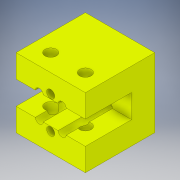
# Autodesk Inventor part: sevo_piece
Saved by Autodesk Inventor 2019 (Build 230136000, 136)
## iProperties
Created: 2019-02-02
Part Number: sevo_piece
Material: Generic
Document SubType Name: Modeling
Designer: suchanek
Density: 1 g/cm^3
Appearance: Default
Author: suchanek
Autodesk Inventor part; units mm, degrees
ref_plane "YZ Plane" through (0, 0, 0) normal (1, 0, 0) x (0, 1, 0)
ref_plane "XZ Plane" through (0, 0, 0) normal (0, 1, 0) x (-1, 0, 0)
ref_plane "XY Plane" through (0, 0, 0) normal (0, 0, 1) x (1, 0, 0)
sketch "Sketch1" plane through (0, 0, 0) normal (0, 0, 1) x (1, 0, 0)
  circle A0 centre (0, 0) radius 10
  circle A1 centre (0, 7) radius 0.85
  circle A2 centre (-4.9497, 4.9497) radius 0.85
  circle A3 centre (-7, 0) radius 0.85
  circle A4 centre (-4.9497, -4.9497) radius 0.85
  circle A5 centre (0, -7) radius 0.85
  circle A6 centre (4.9497, -4.9497) radius 0.85
  circle A7 centre (7, 0) radius 0.85
  circle A8 centre (4.9497, 4.9497) radius 0.85
  dimension "d0" = 20
  dimension "d1" = 7
  dimension "d2" = 1.7
  dimension "d5" = 360
  constraints: 9 centre point, 2 coincident, 1 vertical alignment, 17 other
  measures "d0" diameter of A0
  measures "d1" distance of A1.centre point (0, 0)
  measures "d2" diameter of A1
extrude "Extrusion1" add sketch "Sketch1" along normal blind 14
sketch "Sketch2" plane through (0, 0, 14) normal (0, 0, 1) x (1, 0, 0)
  line L0 (15, -15) -> (-15, -15)
  line L1 (-15, -15) -> (-15, 15)
  line L2 (-15, 15) -> (15, 15)
  line L3 (15, 15) -> (15, -15)
  line L4 (15, -15) -> (-15, 15) construction
  line L5 (-15, -15) -> (15, 15) construction
  point P0 (0, 0)
  dimension "d9" = 30
  dimension "d10" = 30
  constraints: 12 end point, 2 midpoint, 2 parallel, 1 horizontal, 1 perpendicular
  measures "d9" distance of L1.end L2.end
  measures "d10" distance of L0.end L1.end
extrude "Extrusion2" add sketch "Sketch2" against normal blind 10
sketch "Sketch3" plane through (0, 0, 14) normal (0, 0, 1) x (1, 0, 0)
  line L0 (15, 15) -> (15, -15) projected
  line L1 (-15, -15) -> (15, -15)
  line L2 (15, -15) -> (15, -5.1)
  line L3 (15, -5.1) -> (-15, -5.1)
  line L4 (-15, -5.1) -> (-15, -15)
  line L5 (-15, -15) -> (-15, 15) projected
  line L6 (15, 15) -> (-15, 15)
  line L7 (-15, 15) -> (-15, 5.1)
  line L8 (-15, 5.1) -> (15, 5.1)
  line L9 (15, 5.1) -> (15, 15)
  point P0 (0, 0)
  dimension "d13" = 9.9
  dimension "d14" = 9.9
  constraints: 16 end point, 4 parallel, 2 horizontal, 2 perpendicular, 2 point on line
  measures "d13" distance between parallel lines of L1 L3
  measures "d14" distance between parallel lines of L6 L8
extrude "Extrusion3" add sketch "Sketch3" along normal blind 20 contours L0 L8 L5 L6 | L0 L1 L4 L3
sketch "Sketch4" plane through (0, 0, 14) normal (0, 0, 1) x (1, 0, 0)
  point P0 (0, 0)
  point P1 (7, 0)
  point P2 (4.9497, 4.9497)
  point P3 (0, 7)
  point P4 (-4.9497, 4.9497)
  point P5 (-7, 0)
  point P6 (-4.9497, -4.9497)
  point P7 (0, -7)
  point P8 (4.9497, -4.9497)
  dimension "d17" = 7
  dimension "d20" = 360
  constraints: 1 horizontal alignment, 9 other
  measures "d17" distance of point (0, 0) point (7, 0)
hole "Hole1" at (0, -7, 14) at (-4.9497, -4.9497, 14) at (-7, 0, 14) at (4.9497, -4.9497, 14) at (4.9497, 4.9497, 14) at (7, 0, 14) at (-4.9497, 4.9497, 14) at (0, 7, 14) direction (0, 0, -1) diameter 1.8 depth 10 start extended yes counterbore diameter 3.5 counterbore depth 2
sketch "Sketch5" plane through (-15, 15, 4) normal (0, 1, 0) x (1, 0, 0)
  circle A0 centre (7.5, -22.5) radius 2.5
  circle A1 centre (22.5, -22.5) radius 2.5
  line L0 (15, 4) -> (15, -14.6414)
  line L1 (0, -30) -> (0, 0) projected
  line L2 (0, 0) -> (30, 0) projected
  dimension "d29" = 5
  dimension "d30" = 5
  dimension "d32" = 15
  dimension "d33" = 22.5
  constraints: 2 centre point, 2 end point, 1 horizontal alignment, 1 symmetric about line, 1 vertical
  measures "d29" diameter of A0
  measures "d30" diameter of A1
  measures "d32" distance of A1.centre A0.centre
  measures "d33" distance from line of L2 A0.centre
extrude "Extrusion4" cut sketch "Sketch5" against normal through all
body "Solid1"
